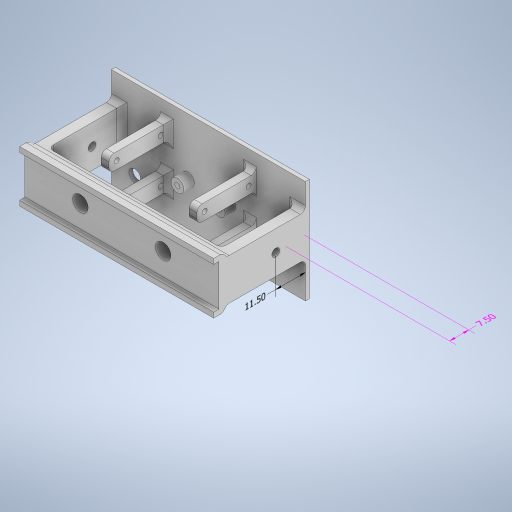
# Autodesk Inventor part: TopCenterElemenV3
Saved by Autodesk Inventor 2024 (Build 280153000, 153)
## iProperties
Created: 2025-03-19
Part Number: TopCenterElemenV3
Material: Ogólny
Document SubType Name: Modeling
Designer: Victoria
Density: 1 g/cm^3
Appearance: Domyślna
Author: Victoria
Autodesk Inventor part; units mm, degrees
ref_plane "YZ Plane" through (0, 0, 0) normal (1, 0, 0) x (0, 1, 0)
ref_plane "XZ Plane" through (0, 0, 0) normal (0, 1, 0) x (-1, 0, 0)
ref_plane "XY Plane" through (0, 0, 0) normal (0, 0, 1) x (1, 0, 0)
sketch "Szkic1" plane through (0, 0, 0) normal (0, 0, 1) x (1, 0, 0)
  line L0 (0, 0) -> (75, 0)
  line L1 (75, 0) -> (75, 45)
  line L2 (75, 45) -> (0, 45)
  line L3 (0, 45) -> (0, 0)
  circle A0 centre (9, 9) radius 2.25
  circle A1 centre (66, 9) radius 2.25
  dimension "d0" = 75
  dimension "d1" = 45
  dimension "d2" = 4.5
  dimension "d3" = 4.5
  dimension "d15" = 9
  dimension "d16" = 9
  dimension "d17" = 9
  dimension "d18" = 9
  constraints: 8 end point, 2 centre point, 2 parallel, 1 horizontal, 1 perpendicular
  measures "d0" distance of L2.end L1.end
  measures "d1" distance of L1.end L0.end
  measures "d2" diameter of A0
  measures "d3" diameter of A1
  measures "d15" distance from line of L3 A0.centre
  measures "d16" distance from line of L0 A0.centre
  measures "d17" distance from line of L1 A1.centre
  measures "d18" distance from line of L0 A1.centre
extrude "Wyciągnięcie proste1" add sketch "Szkic1" along normal blind 1.5
sketch "Szkic10" plane through (0, 0, 1.5) normal (0, 0, 1) x (1, 0, 0)
  line L0 (0, 45) -> (0, 0) projected
  line L1 (0, 30) -> (4, 30)
  line L2 (4, 30) -> (4, 14)
  line L3 (4, 14) -> (0, 14)
  line L4 (0, 14) -> (0, 30)
  line L5 (75, 0) -> (75, 45) projected
  line L6 (75, 30) -> (71, 30)
  line L7 (71, 30) -> (71, 14)
  line L8 (71, 14) -> (75, 14)
  line L9 (75, 14) -> (75, 30)
  point P0 (0, 14)
  dimension "d40" = 4
  dimension "d41" = 16
  dimension "d42" = 4
  dimension "d43" = 16
  constraints: 16 end point, 4 parallel, 2 horizontal, 2 perpendicular, 2 point on line
  measures "d40" distance of L2.end L3.end
  measures "d41" distance of L1.end L2.end
  measures "d42" distance of L8.end L7.end
  measures "d43" distance of L7.end L6.end
extrude "Wyciągnięcie proste10" add sketch "Szkic10" along normal blind 28.5
sketch "Szkic11" plane through (0, 0, 30) normal (0, 0, 1) x (1, 0, 0)
  line L0 (0, 45) -> (0, 30) projected
  line L1 (75, 0) -> (75, 14) projected
  line L2 (0, 30) -> (75, 30)
  line L3 (75, 30) -> (75, 14)
  line L4 (75, 14) -> (0, 14)
  line L5 (0, 14) -> (0, 30)
  point P0 (0, 0)
  constraints: 8 end point, 2 parallel, 1 horizontal, 1 perpendicular
extrude "Wyciągnięcie proste11" add sketch "Szkic11" along normal blind 5
fillet "Zaokrąglenie4" radius 2 8 edges at (4, 22, 30) (4, 22, 1.5) (2, 14, 1.5) (71, 22, 1.5) (73, 14, 1.5) (73, 30, 1.5) (71, 22, 30) (2, 30, 1.5)
sketch "Szkic12" plane through (0, 0, 35) normal (0, 0, 1) x (1, 0, 0)
  circle A0 centre (21.5, 22.7038) radius 3
  line L0 (21.5, 22.7038) -> (53.5, 22.7038)
  line L1 (21.5, 22.7038) -> (53.5, 22.7038) construction
  circle A1 centre (53.5, 22.7038) radius 3
  point P0 (0, 0)
  dimension "d49" = 6
  dimension "d50" = 32
  dimension "d51" = 0
  dimension "d52" = 6
  constraints: 4 end point, 2 centre point, 2 horizontal, 1 coincident, 1 collinear
  measures "d49" diameter of A0
  measures "d50" distance of L0.start L0.end
  measures "d51" distance between parallel lines of L0 L1
  measures "d52" diameter of A1
extrude "Wyciągnięcie proste12" cut sketch "Szkic12" against normal blind 5
sketch "Szkic14" plane through (75, 0, 0) normal (1, 0, 0) x (0, 0, -1)
  circle A0 centre (-9, 22) radius 1.5
  circle A1 centre (-13, 22) radius 1.5
  point P0 (0, 0)
  dimension "d60" = 3
  dimension "d119" = 3
  constraints: 2 centre point
  measures "d60" diameter of A0
  measures "d119" diameter of A1
extrude "Wyciągnięcie proste13" cut sketch "Szkic14" against normal through all contours A1
sketch "Szkic16" plane through (0, 0, 1.5) normal (0, 0, 1) x (1, 0, 0)
  line L0 (19, 33) -> (17, 33) projected
  line L1 (19, 33) -> (22, 33)
  line L2 (22, 33) -> (22, 11)
  line L3 (22, 11) -> (19, 11)
  line L4 (19, 11) -> (19, 33)
  line L5 (56, 0) -> (56, 33) projected
  line L6 (56, 33) -> (53, 33)
  line L7 (53, 33) -> (53, 11)
  line L8 (53, 11) -> (56, 11)
  line L9 (56, 11) -> (56, 33)
  line L10 (19, 33) -> (22, 33)
  line L11 (22, 33) -> (22, 33.5)
  line L12 (22, 33.5) -> (19, 33.5)
  line L13 (19, 33.5) -> (19, 33)
  line L14 (19, 11) -> (22, 11)
  line L15 (22, 11) -> (22, 10.5)
  line L16 (22, 10.5) -> (19, 10.5)
  line L17 (19, 10.5) -> (19, 11)
  line L18 (53, 11) -> (56, 11)
  line L19 (56, 11) -> (56, 10.5)
  line L20 (56, 10.5) -> (53, 10.5)
  line L21 (53, 10.5) -> (53, 11)
  line L22 (53, 33) -> (56, 33)
  line L23 (56, 33) -> (56, 33.5)
  line L24 (56, 33.5) -> (53, 33.5)
  line L25 (53, 33.5) -> (53, 33)
  point P0 (0, 0)
  dimension "d72" = 3
  dimension "d73" = 22
  dimension "d74" = 3
  dimension "d75" = 0.5
  dimension "d76" = 0.5
  dimension "d77" = 0.5
  dimension "d78" = 0.5
  constraints: 48 end point, 12 parallel, 6 horizontal, 6 perpendicular, 4 point on line
  measures "d72" distance of L2.end L3.end
  measures "d73" distance of L1.end L2.end
  measures "d74" distance of L8.end L7.end
  measures "d75" distance of L11.end L10.end
  measures "d76" distance of L14.end L15.end
  measures "d77" distance of L18.end L19.end
  measures "d78" distance of L23.end L22.end
extrude "Wyciągnięcie proste15" add sketch "Szkic16" along normal blind 23
sketch "Szkic18" plane through (56, 10.5, 1.5) normal (1, 0, 0) x (0, 0, -1)
  line L0 (-23, 23) -> (-23, 0) projected
  line L1 (0, 6) -> (-23, 6)
  line L2 (-23, 6) -> (-23, 17)
  line L3 (-23, 17) -> (0, 17)
  line L4 (0, 17) -> (0, 6)
  line L5 (0, 6) -> (-23, 17) construction
  line L6 (-23, 6) -> (0, 17) construction
  circle A0 centre (-20, 3) radius 1
  circle A1 centre (-3, 3) radius 1
  circle A2 centre (-20, 20) radius 1
  circle A3 centre (-3, 20) radius 1
  point P0 (1.5, -10.5)
  point P1 (-11.5, 11.5)
  dimension "d92" = 11
  dimension "d93" = 2
  dimension "d96" = 17
  dimension "d99" = 17
  constraints: 12 end point, 4 centre point, 2 horizontal, 2 midpoint, 2 parallel, 1 perpendicular, 1 point on line, 1 vertical, 6 other
  measures "d92" distance of L1.end L2.end
  measures "d93" diameter of A0
  measures "d96" distance of A0.centre A1.centre
  measures "d99" distance of A0.centre A2.centre
extrude "Wyciągnięcie proste17" cut sketch "Szkic18" against normal up to surface (37 mm away)
fillet "Zaokrąglenie6" radius 2 20 edges at (20.5, 33.5, 1.5) (54.5, 33.5, 1.5) (54.5, 27.5, 24.5) (54.5, 16.5, 24.5) (54.5, 10.5, 24.5) (54.5, 10.5, 1.5) (53, 30.5, 1.5) (53, 13.5, 1.5) (54.5, 16.5, 1.5) (54.5, 27.5, 1.5) (54.5, 33.5, 24.5) (22, 30.5, 1.5) (20.5, 33.5, 24.5) (20.5, 27.5, 24.5) (20.5, 16.5, 24.5) (20.5, 10.5, 24.5) (20.5, 10.5, 1.5) (22, 13.5, 1.5) (20.5, 16.5, 1.5) (20.5, 27.5, 1.5)
sketch "Szkic19" plane through (0, 0, 35) normal (0, 0, 1) x (1, 0, 0)
  line L0 (75, 30) -> (0, 30) projected
  line L1 (75, 0) -> (75, 45) projected
  line L2 (0, 30) -> (75, 30)
  line L3 (75, 30) -> (75, 32)
  line L4 (75, 32) -> (0, 32)
  line L5 (0, 32) -> (0, 30)
  line L6 (75, 14.0293) -> (0, 14.0293)
  line L7 (0, 14.0293) -> (0, 12.0293)
  line L8 (0, 12.0293) -> (75, 12.0293)
  line L9 (75, 12.0293) -> (75, 14.0293)
  point P0 (0, 0)
  dimension "d105" = 2
  dimension "d106" = 2
  constraints: 16 end point, 4 parallel, 3 point on line, 2 horizontal, 2 perpendicular
  measures "d105" distance of L3.end L2.end
  measures "d106" distance of L7.end L6.end
extrude "Wyciągnięcie proste18" add sketch "Szkic19" along normal mid plane 4
fillet "Zaokrąglenie7" radius 2 4 edges at (37.5, 14, 33) (37.5, 12.0293, 33) (37.5, 30, 33) (37.5, 32, 33)
sketch "Szkic20" plane through (0, 0, 1.5) normal (0, 0, 1) x (1, 0, 0)
  line L0 (19, 8.5) -> (19, 18.5) projected
  line L1 (24, 18.5) -> (19, 18.5) projected
  line L2 (24, 8.5) -> (24, 18.5) projected
  line L3 (19, 8.5) -> (24, 8.5) projected
  line L4 (56, 18.5) -> (56, 8.5) projected
  line L5 (51, 8.5) -> (56, 8.5) projected
  line L6 (51, 18.5) -> (51, 8.5) projected
  line L7 (56, 18.5) -> (51, 18.5) projected
  line L8 (56, 35.5) -> (56, 25.5) projected
  line L9 (51, 25.5) -> (56, 25.5) projected
  line L10 (51, 35.5) -> (51, 25.5) projected
  line L11 (56, 35.5) -> (51, 35.5) projected
  line L12 (19, 25.5) -> (19, 35.5) projected
  line L13 (24, 35.5) -> (19, 35.5) projected
  line L14 (24, 25.5) -> (24, 35.5) projected
  line L15 (19, 25.5) -> (24, 25.5) projected
  line L16 (69, 12) -> (75, 12) projected
  line L17 (69, 32) -> (69, 12) projected
  line L18 (75, 32) -> (69, 32) projected
  line L19 (75, 32) -> (75, 45) projected
  line L20 (75, 45) -> (0, 45) projected
  line L21 (0, 45) -> (0, 32) projected
  line L22 (6, 12) -> (6, 32) projected
  line L23 (0, 12) -> (6, 12) projected
  line L24 (0, 12) -> (0, 0) projected
  line L25 (0, 0) -> (75, 0) projected
  line L26 (75, 0) -> (75, 12) projected
  circle A0 centre (9, 9) radius 2.25 projected
  circle A1 centre (66, 9) radius 2.25 projected
  circle A2 centre (45.5, 27.5) radius 1
  circle A3 centre (29.5, 27.5) radius 1
  circle A4 centre (45.5, 27.5) radius 2.5
  circle A5 centre (29.5, 27.5) radius 2.5
  line L27 (6, 32) -> (0, 32) projected
  circle A6 centre (21.5, 22.7038) radius 3 projected
  circle A7 centre (53.5, 22.7038) radius 3 projected
  line L28 (21.5, 22.7038) -> (53.5, 22.7038)
  line L29 (29.5, 27.5) -> (29.5, 17.908)
  circle A8 centre (29.5, 17.908) radius 1
  circle A9 centre (29.5, 17.908) radius 2.5
  circle A10 centre (45.5, 17.908) radius 1
  circle A11 centre (45.5, 17.908) radius 2.5
  dimension "d113" = 2
  dimension "d114" = 2
  dimension "d115" = 1.5
  dimension "d116" = 1.5
  dimension "d122" = 9.592
  dimension "d123" = 2
  dimension "d125" = 1.5
  dimension "d126" = 2
  dimension "d127" = 1.5
  constraints: 8 centre point, 4 end point, 1 coincident, 1 horizontal, 1 perpendicular
  measures "d113" diameter of A2
  measures "d114" diameter of A3
  measures "d115" radial gap between concentric circles of A2 A4
  measures "d116" radial gap between concentric circles of A3 A5
  measures "d122" distance of L29.start L29.end
  measures "d123" diameter of A8
  measures "d125" radial gap between concentric circles of A8 A9
  measures "d126" diameter of A10
  measures "d127" radial gap between concentric circles of A10 A11
extrude "Wyciągnięcie proste19" add sketch "Szkic20" along normal blind 4 contours A9 | A11
sketch "Szkic23" plane through (0, 0, 1.5) normal (0, 0, 1) x (1, 0, 0)
  line L0 (75, 45) -> (0, 45) projected
  line L1 (75, 0) -> (75, 45) projected
  line L2 (0, 45) -> (75, 45)
  line L3 (75, 45) -> (75, 40)
  line L4 (75, 40) -> (0, 40)
  line L5 (0, 40) -> (0, 45)
  point P0 (0, 0)
  dimension "d131" = 5
  constraints: 8 end point, 2 parallel, 1 horizontal, 1 perpendicular, 1 point on line
  measures "d131" distance of L2.end L3.end
extrude "Wyciągnięcie proste21" cut sketch "Szkic23" against normal blind 45
